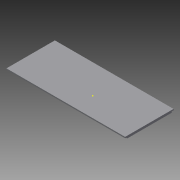
# Autodesk Inventor part: Side
Saved by Autodesk Inventor 2015 (Build 190159000, 159)
## iProperties
Created: 2018-04-13
Part Number: Side
Material: Generic
Document SubType Name: Modeling
Designer: Toby
Density: 1 g/cm^3
Appearance: Default
Author: Toby
Autodesk Inventor part; units mm, degrees
ref_plane "YZ Plane" through (0, 0, 0) normal (1, 0, 0) x (0, 1, 0)
ref_plane "XZ Plane" through (0, 0, 0) normal (0, 1, 0) x (-1, 0, 0)
ref_plane "XY Plane" through (0, 0, 0) normal (0, 0, 1) x (1, 0, 0)
sketch "Sketch1" plane through (0, 0, 0) normal (0, 0, 1) x (1, 0, 0)
  line L0 (-67.8347, 27.5702) -> (52.1653, 27.5702)
  line L1 (52.1653, 27.5702) -> (52.1653, -17.4298)
  line L2 (52.1653, -17.4298) -> (-67.8347, -17.4298)
  line L3 (-67.8347, -17.4298) -> (-67.8347, 27.5702)
  point P0 (0, 0)
  dimension "d0" = 120
  dimension "d1" = 45
  constraints: 8 end point, 2 parallel, 1 horizontal, 1 perpendicular
  measures "d0" distance of L0.start L0.end
  measures "d1" distance of L2.end L0.start
extrude "Extrusion1" add sketch "Sketch1" along normal blind 1.2
sketch "Sketch2" plane through (0, 0, 1.2) normal (0, 0, 1) x (1, 0, 0)
  line L0 (-67.8347, 29.5702) -> (52.1653, 29.5702)
  line L1 (52.1653, 29.5702) -> (52.1653, -19.4298)
  line L2 (52.1653, -19.4298) -> (-67.8347, -19.4298)
  line L3 (-67.8347, -19.4298) -> (-67.8347, 29.5702)
  line L4 (52.1653, 27.5702) -> (-67.8347, 27.5702) projected
  line L5 (52.1653, -17.4298) -> (-67.8347, -17.4298) projected
  line L6 (-67.8347, 27.5702) -> (-67.8347, -17.4298) projected
  line L7 (52.1653, -17.4298) -> (52.1653, 27.5702) projected
  point P0 (0, 0)
  dimension "d4" = 2
  dimension "d5" = 2
  constraints: 8 end point, 2 collinear, 2 parallel, 1 horizontal, 1 perpendicular
  measures "d4" distance between parallel lines of L4 L0
  measures "d5" distance between parallel lines of L5 L2
extrude "Extrusion2" add sketch "Sketch2" along normal blind 1.2
sketch "Sketch3" plane through (0, 0, 2.4) normal (0, 0, 1) x (1, 0, 0)
  point P0 (0, 0)
body "Solid1"
